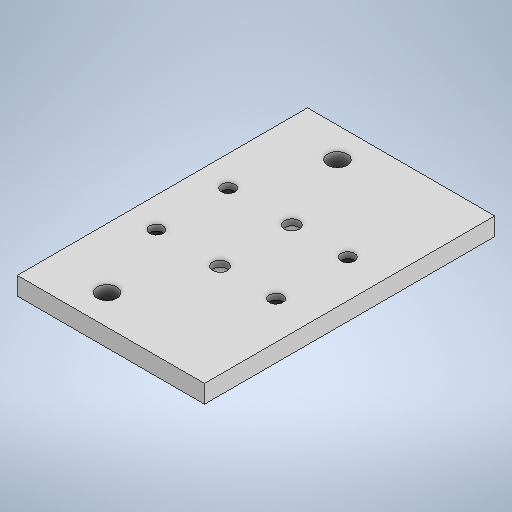
# Autodesk Inventor part: TS_Halterung_Fuehrungszylinder_int
Saved by Autodesk Inventor 2025.2 (Build 292293000, 293)
## iProperties
Created: 2025-06-19
Part Number: TS_Halterung_Fuehrungszylinder_int
Material: Generisch
Document SubType Name: Modeling
Designer: tino
Density: 1 g/cm^3
Appearance: Vorgabe
Author: tino
Autodesk Inventor part; units mm, degrees
ref_plane "YZ Plane" through (0, 0, 0) normal (1, 0, 0) x (0, 1, 0)
ref_plane "XZ Plane" through (0, 0, 0) normal (0, 1, 0) x (-1, 0, 0)
ref_plane "XY Plane" through (0, 0, 0) normal (0, 0, 1) x (1, 0, 0)
sketch "Skizze1" plane through (0, 0, 0) normal (0, 0, 1) x (1, 0, 0)
  line L0 (-31.2875, 48.5) -> (31.2875, 48.5)
  line L1 (31.2875, 48.5) -> (31.2875, -48.5)
  line L2 (31.2875, -48.5) -> (-31.2875, -48.5)
  line L3 (-31.2875, -48.5) -> (-31.2875, 48.5)
  line L4 (-31.2875, 48.5) -> (31.2875, -48.5) construction
  line L5 (31.2875, 48.5) -> (-31.2875, -48.5) construction
  point P0 (0, 0)
  point P1 (-21.2875, -12)
  point P2 (18.7125, -12)
  point P3 (18.7125, 12)
  point P4 (-21.2875, 12)
  dimension "d0" = 62.575
  dimension "d1" = 97
  dimension "d2" = 52.575
  dimension "d3" = 40
  dimension "d18" = 12
  dimension "d19" = 24
  constraints: 12 end point, 2 horizontal alignment, 2 midpoint, 2 parallel, 2 vertical alignment, 1 horizontal, 1 perpendicular
  measures "d0" distance of L0.start L0.end
  measures "d1" distance of L0.end L1.end
  measures "d2" distance from line of L1 point (-21.288, -12)
  measures "d3" distance of point (18.712, -12) point (-21.288, -12)
  measures "d18" vertical distance of point (18.712, 12) point (0, 0)
  measures "d19" distance of point (18.712, 12) point (18.712, -12)
extrude "Extrusion1" add sketch "Skizze1" along normal blind 6
sketch "Skizze2" plane through (0, 0, 0) normal (0, 0, -1) x (-1, 0, 0)
  line L0 (31.2875, 48.5) -> (31.2875, -48.5) projected
  point P0 (21.2875, -12)
  point P1 (-18.7125, -12)
  point P2 (0, 0)
  point P3 (-18.7125, 12)
  point P4 (21.2875, 12)
  point P5 (-18.7125, -12)
  dimension "d9" = 40
  dimension "d10" = 10
  dimension "d20" = 24
  dimension "d21" = 12
  constraints: 2 horizontal alignment, 2 vertical alignment, 1 coincident
  measures "d9" distance of point (-18.713, -12) point (21.287, -12)
  measures "d10" distance from line of L0 point (21.287, -12)
  measures "d20" distance of point (-18.713, 12) point (-18.713, -12)
  measures "d21" vertical distance of point (0, 0) point (-18.713, 12)
hole "Bohrung1" at (-21.2875, -12, 0) at (18.7125, -12, 0) at (18.7125, 12, 0) at (-21.2875, 12, 0) direction (0, 0, 1) diameter 4.5 end through all counterbore diameter 8 counterbore depth 4 clearance for "Innensechskantkopfschraube" size "M4" standard "ANSI Metrisches M Profil"
sketch "Skizze3" plane through (0, 0, 6) normal (0, 0, 1) x (1, 0, 0)
  circle A0 centre (18.7125, -12) radius 2.25 projected
  circle A1 centre (-21.2875, -12) radius 2.25 projected
  circle A2 centre (-21.2875, 12) radius 2.25 projected
  circle A3 centre (18.7125, 12) radius 2.25 projected
  point P0 (0, 0)
  point P1 (0, -12)
  point P2 (0, 12)
  constraints: 2 horizontal alignment, 2 vertical alignment
hole "Bohrung2" at (0, -12, 6) at (0, 12, 6) direction (0, 0, -1) diameter 5 depth 2
sketch "Skizze4" plane through (0, 0, 6) normal (0, 0, 1) x (1, 0, 0)
  line L0 (-31.2875, -48.5) -> (31.2875, -48.5) projected
  line L1 (31.2875, 48.5) -> (-31.2875, 48.5) projected
  line L2 (-31.2875, 48.5) -> (-31.2875, -48.5) projected
  point P0 (0, 0)
  point P1 (-11.2875, -38.5)
  point P2 (-11.2875, 38.5)
  dimension "d29" = 10
  dimension "d30" = 10
  dimension "d31" = 20
  constraints: 1 vertical alignment
  measures "d29" distance from line of L0 point (-11.287, -38.5)
  measures "d30" distance from line of L1 point (-11.287, 38.5)
  measures "d31" distance from line of L2 point (-11.287, -38.5)
hole "Bohrung3" at (-11.2875, -38.5, 6) at (-11.2875, 38.5, 6) direction (0, 0, -1) diameter 6.6 end through all clearance for "Innensechskantkopfschraube" size "M6" standard "ANSI Metrisches M Profil"
